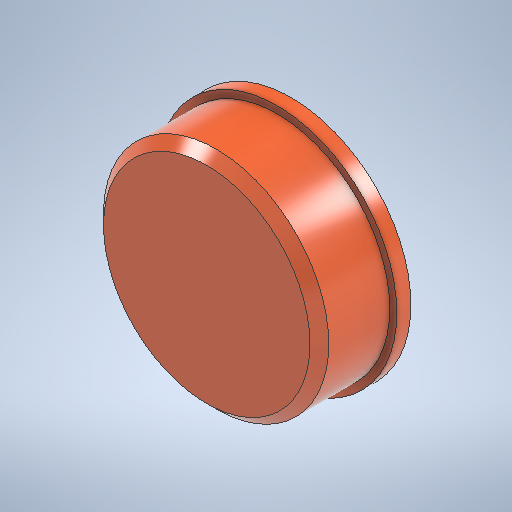
# Autodesk Inventor part: botão final
Saved by Autodesk Inventor 2025 (Build 290162000, 162)
## iProperties
Created: 2026-05-19
Part Number: botão final
Material: Genérico
Document SubType Name: Modeling
Designer: pedro
Density: 1 g/cm^3
Appearance: Padrão
Author: pedro
Autodesk Inventor part; units mm, degrees
ref_plane "YZ Plane" through (0, 0, 0) normal (1, 0, 0) x (0, 1, 0)
ref_plane "XZ Plane" through (0, 0, 0) normal (0, 1, 0) x (-1, 0, 0)
ref_plane "XY Plane" through (0, 0, 0) normal (0, 0, 1) x (1, 0, 0)
sketch "Esboço1" plane through (0, 0, 0) normal (0, 0, 1) x (1, 0, 0)
  circle A0 centre (0, 0) radius 2.4
  dimension "d0" = 4.8
  constraints: 1 centre point, 1 coincident
  measures "d0" diameter of A0
extrude "Extrusão1" add sketch "Esboço1" along normal blind 1.5
sketch "Esboço2" plane through (0, 0, 0) normal (0, 0, -1) x (-1, 0, 0)
  circle A0 centre (0, 0) radius 2.55
  dimension "d3" = 5.1
  constraints: 1 centre point, 1 coincident
  measures "d3" diameter of A0
extrude "Extrusão2" add sketch "Esboço2" along normal blind 0.3
sketch "Esboço4" plane through (0, 0, -0.3) normal (0, 0, -1) x (-1, 0, 0)
  line L0 (-0.5, 2) -> (0.5, 2)
  line L1 (0.5, 2) -> (0.5, -2)
  line L2 (0.5, -2) -> (-0.5, -2)
  line L3 (-0.5, -2) -> (-0.5, 2)
  line L4 (-2, 0.5) -> (2, 0.5)
  line L5 (2, 0.5) -> (2, -0.5)
  line L6 (2, -0.5) -> (-2, -0.5)
  line L7 (-2, -0.5) -> (-2, 0.5)
  point P0 (0, 0)
  point P1 (-2, 0)
  point P2 (0, 0.5)
  point P3 (0, 2)
  point P4 (0.5, 0)
  point P5 (-0.5, 0.5)
  point P6 (-0.5, -0.5)
  point P7 (0.5, -0.5)
  point P8 (0.5, 0.5)
  dimension "d6" = 1
  dimension "d7" = 4
  dimension "d8" = 4
  dimension "d9" = 1
  constraints: 16 end point, 4 midpoint, 4 parallel, 2 horizontal, 2 horizontal alignment, 2 perpendicular, 2 vertical alignment
  measures "d6" distance of L1.end L2.end
  measures "d7" distance of L0.end L1.end
  measures "d8" distance of L5.end L6.end
  measures "d9" distance of L4.end L5.end
extrude "Extrusão3" add sketch "Esboço4" along normal blind 0.3 and the other way blind 0.3
chamfer "Chanfro1" distance 0.2 angle 45 1 edges at (-2.4, 0, 1.5)
